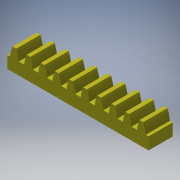
# Autodesk Inventor part: МД.001.1003 - Рейка
Saved by Autodesk Inventor 2019 (Build 230136000, 136)
## iProperties
Created: 2019-12-30
Part Number: МД.001.1003 - Рейка
Material: Пластик АБС
Document SubType Name: Modeling
Designer: Петров Иван
Density: 1.06 g/cm^3
Appearance: Канареечный
Author: Петров Иван
Autodesk Inventor part; units mm, degrees
ref_plane "YZ Plane" through (0, 0, 0) normal (1, 0, 0) x (0, 1, 0)
ref_plane "XZ Plane" through (0, 0, 0) normal (0, 1, 0) x (-1, 0, 0)
ref_plane "XY Plane" through (0, 0, 0) normal (0, 0, 1) x (1, 0, 0)
sketch "Эскиз3" plane through (0, 0, 0) normal (0, 0, 1) x (1, 0, 0)
  arc A0 (-0.3052, 6.9905) -> (-0.7081, 5.3786) centre (4.7456, 4.8717) ccw
  arc A1 (0.3052, 6.9905) -> (-0.3052, 6.9905) centre (0, 0) ccw
  arc A2 (0.7081, 5.3786) -> (0.3052, 6.9905) centre (-4.7456, 4.8717) ccw
  line L0 (-0.7081, 5.3786) -> (-1.1742, 5.3786)
  line L1 (1.1742, 5.3786) -> (1.1742, 3.3786)
  line L2 (1.1742, 3.3786) -> (-1.1742, 3.3786)
  line L3 (-1.1742, 3.3786) -> (-1.1742, 5.3786)
  line L4 (-1.1742, 5.3786) -> (-0.7081, 5.3786)
  line L5 (0.7081, 5.3786) -> (1.1742, 5.3786)
  line L6 (-1.1742, 5.3786) -> (-0.7081, 5.3786)
  line L7 (0.7081, 5.3786) -> (1.1742, 5.3786)
  dimension "d9" = 2
  constraints: 16 end point, 6 point on circle, 3 centre point, 3 horizontal, 3 parallel, 2 perpendicular, 1 point on line
  measures "d9" distance of L1.start L1.end
extrude "Выдавливание4" add sketch "Эскиз3" along normal blind 4
pattern_linear "Прямоуг.массив2" count 10 spacing 2.33 along (1, 0, 0) of "Выдавливание4"
equation "\"Модуль\" = 0.7"
equation "\"Угол_зацепления\" = 20deg"
equation "\"Зазор_профиля_зуба\" = 0.25"
equation "\"Радиус_закругления_зуба\" = 0.35"
equation "\"Диаметр_головки\" = 19.87688"
equation "\"Диаметр_впадин\" = 16.73076"
equation "\"Основной_диаметр\" = 17.33474"
equation "\"Средний_диаметр\" = 18.48076"
equation "\"Ширина_грани\" = 4"
equation "\"Коэффициент_смещения\" = 0"
equation "\"Изменение_высоты_головки_зуба\" = 0.002778"
equation "\"Окружной_шаг\" = 2.23304"
equation "\"Общий_сдвиг_инструмента\" = 0"
equation "\"Внутренний\" = 0"
